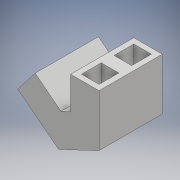
# Autodesk Inventor part: backwheel_Cap
Saved by Autodesk Inventor 2018.3 (Build 223284000, 284)
## iProperties
Created: 2020-10-24
Part Number: backwheel_Cap
Material: Generic
Document SubType Name: Modeling
Designer: chris
Density: 1 g/cm^3
Appearance: Default
Author: chris
Autodesk Inventor part; units mm, degrees
ref_plane "YZ Plane" through (0, 0, 0) normal (1, 0, 0) x (0, 1, 0)
ref_plane "XZ Plane" through (0, 0, 0) normal (0, 1, 0) x (-1, 0, 0)
sketch "Sketch1" plane through (0, 0, 0) normal (0, 0, 1) x (1, 0, 0)
  line L0 (19.1, 20.9) -> (4.5, 20.9) construction
  line L1 (19.1, 20.9) -> (19.1, 4.5) construction
  line L2 (19.1, 4.5) -> (4.5, 4.5) construction
  line L3 (4.5, 4.5) -> (4.5, 20.9) construction
  line L4 (4.5, 47.9069) -> (4.5, 31.5069) construction
  line L5 (19.1, 47.9069) -> (4.5, 47.9069) construction
  line L6 (19.1, 31.5069) -> (19.1, 47.9069) construction
  line L7 (4.5, 31.5069) -> (19.1, 31.5069) construction
  line L8 (0, 0) -> (0, 52.4069) construction
  line L9 (0, 0) -> (23.6, 0) construction
  line L10 (23.6, 0) -> (23.6, 52.4069) construction
  line L11 (0, 52.4069) -> (23.6, 52.4069) construction
  line L12 (0, 52.4069) -> (0, 0) construction
  line L13 (23.6, 0) -> (23.6, 52.4069) construction
  line L14 (0, 52.4069) -> (23.6, 52.4069)
  line L15 (23.6, 52.4069) -> (23.6, 0)
  line L16 (23.6, 0) -> (0, 0)
  line L17 (0, 0) -> (0, 52.4069)
  line L18 (4.5, 4.5) -> (4.5, 20.9) construction
  line L19 (19.1, 20.9) -> (19.1, 4.5) construction
  line L20 (4.5, 20.9) -> (19.1, 20.9)
  line L21 (19.1, 20.9) -> (19.1, 4.5)
  line L22 (19.1, 4.5) -> (4.5, 4.5)
  line L23 (4.5, 4.5) -> (4.5, 20.9)
  line L24 (4.5, 47.9069) -> (19.1, 47.9069)
  line L25 (19.1, 47.9069) -> (19.1, 31.5069)
  line L26 (19.1, 31.5069) -> (4.5, 31.5069)
  line L27 (4.5, 31.5069) -> (4.5, 47.9069)
  point P0 (0, 0)
  point P1 (-49.87, 37.7316)
  constraints: 56 end point, 6 parallel, 3 horizontal, 3 perpendicular
extrude "Extrusion1" add sketch "Sketch1" along normal blind 40
sketch "Sketch2" plane through (0, 52.4069, 0) normal (0, 1, 0) x (1, 0, 0)
  line L0 (0, 0) -> (23.6, 0) construction
  line L1 (0, 0) -> (0, -40) construction
  line L2 (23.6, -40) -> (0, -40) construction
  line L3 (23.6, 0) -> (23.6, -40) construction
  line L4 (4.5, 0) -> (-0.53, 0)
  line L5 (4.5, 0) -> (9.53, 0) construction
  line L6 (-0.53, 0) -> (-0.53, 2.023)
  line L7 (-0.53, 0) -> (1.493, 0) construction
  constraints: 8 end point, 2 equal length, 2 horizontal, 1 coincident, 1 collinear, 1 vertical
ref_plane "Work Plane1" through (-0.53, 52.4069, -2.023) normal (-0.790155, 0, 0.6129071) x (0, 1, 0)
sketch "Sketch3" plane through (-0.53, 52.4069, -2.023) normal (-0.790155, 0, 0.6129071) x (0, 1, 0)
  line L0 (-20.9, 14.6) -> (-20.9, 0) construction
  line L1 (-20.9, 14.6) -> (-4.5, 14.6) construction
  line L2 (-4.5, 14.6) -> (-4.5, 0) construction
  line L3 (-4.5, 0) -> (-20.9, 0) construction
  line L4 (-47.9069, 0) -> (-31.5069, 0) construction
  line L5 (-47.9069, 14.6) -> (-47.9069, 0) construction
  line L6 (-31.5069, 14.6) -> (-47.9069, 14.6) construction
  line L7 (-31.5069, 0) -> (-31.5069, 14.6) construction
  line L8 (0, -4.5) -> (-52.4069, -4.5) construction
  line L9 (0, -4.5) -> (0, 19.1) construction
  line L10 (0, 19.1) -> (-52.4069, 19.1) construction
  line L11 (-52.4069, -4.5) -> (-52.4069, 19.1) construction
  line L12 (-52.4069, -4.5) -> (0, -4.5) construction
  line L13 (0, 19.1) -> (-52.4069, 19.1) construction
  line L14 (-52.4069, -4.5) -> (-52.4069, 19.1)
  line L15 (-52.4069, 19.1) -> (0, 19.1)
  line L16 (0, 19.1) -> (0, -4.5)
  line L17 (0, -4.5) -> (-52.4069, -4.5)
  line L18 (-4.5, 0) -> (-20.9, 0) construction
  line L19 (-20.9, 14.6) -> (-4.5, 14.6) construction
  line L20 (-20.9, 0) -> (-20.9, 14.6)
  line L21 (-20.9, 14.6) -> (-4.5, 14.6)
  line L22 (-4.5, 14.6) -> (-4.5, 0)
  line L23 (-4.5, 0) -> (-20.9, 0)
  line L24 (-47.9069, 0) -> (-47.9069, 14.6)
  line L25 (-47.9069, 14.6) -> (-31.5069, 14.6)
  line L26 (-31.5069, 14.6) -> (-31.5069, 0)
  line L27 (-31.5069, 0) -> (-47.9069, 0)
  point P0 (-52.4069, -1.9233)
  point P1 (-49.87, 37.7316)
  point P2 (-4.5, 0)
  constraints: 56 end point, 6 parallel, 3 perpendicular
extrude "Extrusion2" add sketch "Sketch3" along normal blind 40
sketch "Sketch4" plane through (0, 52.4069, 40) normal (0, 1, 0) x (1, 0, 0)
  line L0 (-12.2365, 57.115) -> (-43.8427, 32.5987) construction
  line L1 (1.0392, 40) -> (23.6, 40) construction
  line L2 (23.6, 40) -> (23.6, 43)
  line L3 (23.6, 40) -> (26.6, 40) construction
  line L4 (-12.2365, 57.115) -> (-9.8661, 58.9537)
  line L5 (-9.8661, 58.9537) -> (23.6, 43)
  line L6 (1.0392, 40) -> (-12.2365, 57.115) construction
  line L7 (-12.2365, 57.115) -> (1.0392, 40)
  line L8 (23.6, 40) -> (1.0392, 40) construction
  line L9 (1.0392, 40) -> (23.6, 40)
  point P0 (0, 40)
  point P1 (4.5, 40)
  point P2 (-0.53, 42.023)
  dimension "d9" = 3
  dimension "d10" = 90
  dimension "d11" = 3
  constraints: 12 end point, 2 collinear, 1 horizontal, 1 perpendicular, 1 point on line, 1 vertical
  measures "d9" distance of L1.end L2.end
  measures "d10" angle of L3 L2
  measures "d11" distance of L0.start L4.end
extrude "Extrusion3" add sketch "Sketch4" against normal up to surface (52.4069 mm away)
sketch "Sketch5" plane through (0, 52.4069, 40) normal (0, 1, 0) x (1, 0, 0)
  line L0 (-9.8661, 58.9537) -> (23.6, 43) construction
  line L1 (0, 36.739) -> (0, 0) construction
  line L2 (0, 36.739) -> (0, 26.739)
  line L3 (0, 26.739) -> (-7.9847, 30.5454)
  line L4 (0, 36.739) -> (-7.9847, 30.5454)
  line L5 (0, 36.739) -> (-29.3781, 13.951) construction
  point P0 (0, 40)
  constraints: 6 end point, 2 point on line, 1 parallel
extrude "Extrusion4" add sketch "Sketch5" against normal up to surface (52.4069 mm away)
body "Solid1"
